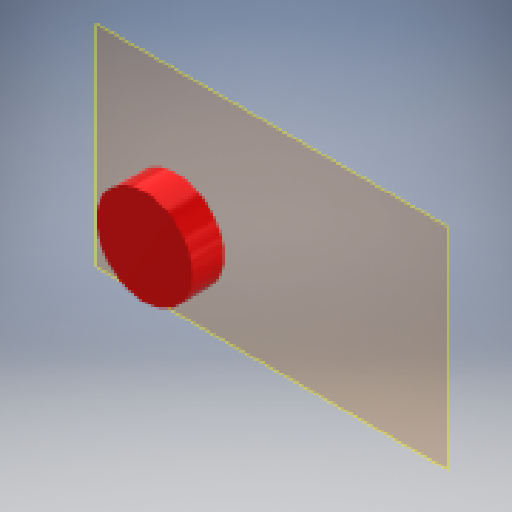
# Autodesk Inventor part: CE-8.2.2-01-002
Saved by Autodesk Inventor 2024 (Build 280153000, 153)
## iProperties
Created: 2024-03-07
Part Number: CE-8.2.2-01-002
Material: Generic
Document SubType Name: Modeling
Designer: Alex
Density: 1 g/cm^3
Appearance: Red
Author: Alex
Autodesk Inventor part; units mm, degrees
ref_plane "YZ Plane" through (0, 0, 0) normal (1, 0, 0) x (0, 1, 0)
ref_plane "XZ Plane" through (0, 0, 0) normal (0, 1, 0) x (-1, 0, 0)
ref_plane "XY Plane" through (0, 0, 0) normal (0, 0, 1) x (1, 0, 0)
ref_plane "Work Plane1" through (47.8715, -11.8355, -36.036) normal (0, 0, 1) x (1, 0, 0)
sketch "Sketch1" plane through (47.8715, -11.8355, -36.036) normal (0, 0, 1) x (1, 0, 0)
  circle A0 centre (40, 40) radius 30
  point P0 (-47.8715, 11.8355)
  constraints: 1 centre point, 2 other
extrude "Extrusion1" add sketch "Sketch1" along normal blind 20
body "Solid1"
